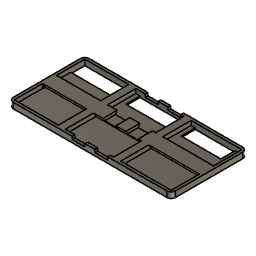
Top Side Cover 3x1 v5 (Autodesk Fusion 360 design; units mm, degrees)
Autodesk Fusion 360 part; units mm, degrees
sketch "Schizzo1" plane through (0, 0, 0) normal (0, 0, 1) x (1, 0, 0)
  line L0 (4.5367, 58.7959) -> (119.2367, 58.7959) construction
  line L1 (119.2367, 58.7959) -> (119.2367, 5.0959) construction
  line L2 (119.2367, 5.0959) -> (4.5367, 5.0959) construction
  line L3 (4.5367, 5.0959) -> (4.5367, 58.7959) construction
  line L4 (4.5367, 31.9459) -> (119.2367, 31.9459) construction
  line L5 (61.8867, 58.7959) -> (61.8867, 5.0959) construction
  line L6 (119.1367, 5.1959) -> (4.6367, 5.1959)
  line L7 (4.6367, 5.1959) -> (4.6367, 58.6959)
  line L8 (4.6367, 58.6959) -> (119.1367, 58.6959)
  line L9 (119.1367, 58.6959) -> (119.1367, 5.1959)
  line L10 (117.2367, 7.0959) -> (6.5367, 7.0959)
  line L11 (6.5367, 7.0959) -> (6.5367, 56.7959)
  line L12 (6.5367, 56.7959) -> (117.2367, 56.7959)
  line L13 (117.2367, 56.7959) -> (117.2367, 7.0959)
  line L14 (6.5367, 56.7959) -> (34.5367, 56.7959)
  line L15 (34.5367, 56.7959) -> (34.5367, 46.7959)
  line L16 (34.5367, 46.7959) -> (6.5367, 46.7959)
  line L17 (6.5367, 46.7959) -> (6.5367, 56.7959)
  line L18 (73.5367, 56.7959) -> (73.5367, 46.7959)
  line L19 (73.5367, 46.7959) -> (45.5367, 46.7959)
  line L20 (45.5367, 46.7959) -> (45.5367, 56.7959)
  line L21 (45.5367, 56.7959) -> (73.5367, 56.7959)
  line L22 (4.5367, 36.9459) -> (119.1367, 36.9459)
  line L23 (4.5367, 26.9459) -> (119.1367, 26.9459)
  line L24 (61.8867, 58.7959) -> (61.8867, 5.0959)
  line L25 (112.5367, 56.7959) -> (112.5367, 46.7959)
  line L26 (112.5367, 46.7959) -> (84.5367, 46.7959)
  line L27 (84.5367, 46.7959) -> (84.5367, 56.7959)
  line L28 (84.5367, 56.7959) -> (112.5367, 56.7959)
  line L29 (37.5367, 58.7959) -> (37.5367, 5.0959)
  line L30 (42.5367, 58.7959) -> (42.5367, 5.0959)
  line L31 (76.5367, 58.7959) -> (76.5367, 5.0959)
  line L32 (81.5367, 58.6959) -> (81.5367, 5.0959)
  dimension "d1" = 114.7
  dimension "d2" = 53.7
  dimension "d3" = 0.1
  dimension "d6" = 2
  dimension "d7" = 28
  dimension "d8" = 10
  dimension "d11" = 39
  dimension "d12" = 0
  dimension "d15" = 10
  dimension "d38" = 5
  dimension "d39" = 3
  dimension "d40" = 5
  dimension "d41" = 3
  constraint horizontal L0
  constraint vertical L1
  constraint horizontal L2
  constraint vertical L3
  constraint midpoint L3 L4.start
  constraint midpoint L1 L4.end
  constraint midpoint L0 L5.start
  constraint midpoint L2 L5.end
  constraint horizontal L14
  constraint vertical L15
  constraint horizontal L16
  constraint vertical L17
  constraint coincident L3 L22.start
  constraint coincident L9 L22.end
  constraint perpendicular L9 L22
  constraint symmetric L4 L22.start L23.start
  constraint symmetric L4 L22.end L23.end
  constraint coincident L0 L29.start
  constraint coincident L2 L29.end
  constraint perpendicular L6 L29
  constraint coincident L0 L30.start
  constraint coincident L2 L30.end
  constraint perpendicular L6 L30
  constraint coincident L0 L31.start
  constraint coincident L2 L31.end
  constraint perpendicular L2 L31
  constraint coincident L8 L32.start
  constraint coincident L2 L32.end
  constraint perpendicular L6 L32
  measures "d1" distance of L1 L3
  measures "d2" distance of L0 L2
  measures "d7" distance of L11.end L14.end
  measures "d8" distance of L11.end L16.end
  measures "d15" distance of L22 L23
  measures "d38" distance of L29 L30
  measures "d39" distance of L20 L30
  measures "d40" distance of L31 L32
  measures "d41" distance of L18 L31
extrude "Estrusione1" add sketch "Schizzo1" along normal blind 1 contours L10 L13 L23 L32 | L10 L23 L31 L32 | L13 L22 L23 L32 | L10 L23 L24 L31 | L22 L23 L31 L32 | L12 L13 L22 L25 L26 L27 L32 | L10 L23 L24 L30 | L22 L23 L24 L31 | L12 L22 L31 L32 | L10 L23 L29 L30 | L22 L23 L24 L30 | L12 L18 L19 L22 L24 L31 | L10 L11 L23 L29 | L22 L23 L29 L30 | L12 L19 L20 L22 L24 L30 | L11 L22 L23 L29 | L12 L22 L29 L30 | L11 L12 L15 L16 L22 L29
extrude "Estrusione2" add sketch "Schizzo1" along normal blind 4 contours L6 L9 L10 L13 L23 L32 | L6 L10 L31 L32 | L9 L13 L22 L23 | L6 L10 L24 L31 | L8 L9 L12 L13 L22 L28 L32 | L13 L22 L23 L32 | L6 L10 L24 L30 | L22 L23 L31 L32 | L6 L10 L29 L30 | L22 L23 L24 L31 | L8 L12 L31 L32 | L6 L7 L10 L11 L23 L29 | L22 L23 L24 L30 | L8 L12 L21 L24 L31 | L22 L23 L29 L30 | L8 L12 L21 L24 L30 | L7 L11 L22 L23 | L11 L22 L23 L29 | L8 L12 L29 L30 | L7 L8 L11 L12 L14 L17 L22 L29
fillet "Raccordo1" radius 3 4 edges at (4.6367, 5.1959, 2) (119.1367, 5.1959, 2) (119.1367, 58.6959, 2) (4.6367, 58.6959, 2)
ref_plane "Piano di lavoro1" through (61.8867, 31.9459, 0) normal (-1, 0, 0) x (0, -1, 0)
sketch "Schizzo3" plane through (61.8867, 0, 0) normal (-1, 0, 0) x (0, -1, 0)
  line L0 (-26.9459, 4) -> (-36.9459, 4) construction
  line L1 (-36.9459, 4) -> (-36.9459, 0) construction
  line L2 (-36.9459, 0) -> (-26.9459, 0) construction
  line L3 (-26.9459, 0) -> (-26.9459, 4) construction
  line L4 (-55.6959, 4) -> (-8.1959, 4) construction
  line L5 (-58.7959, 0) -> (-5.0959, 0) construction
  line L6 (-26.9459, 1) -> (-26.9459, 4) construction
  line L7 (-36.9459, 1) -> (-36.9459, 4) construction
  line L8 (-31.9459, 4) -> (-31.9459, 0) construction
  line L9 (-26.9459, 1) -> (-36.9459, 1) construction
  line L10 (-26.9459, 1) -> (-26.9459, 4)
  line L11 (-26.9459, 4) -> (-28.678, 1)
  line L12 (-28.678, 1) -> (-26.9459, 1)
  line L13 (-36.9459, 1) -> (-36.9459, 4)
  line L14 (-36.9459, 4) -> (-35.2139, 1)
  line L15 (-35.2139, 1) -> (-36.9459, 1)
  dimension "d20" = 30
  constraint horizontal L0
  constraint vertical L1
  constraint horizontal L2
  constraint vertical L3
  constraint collinear L0 L4
  constraint collinear L2 L5
  constraint collinear L3 L6
  constraint collinear L1 L7
  constraint midpoint L4 L8.start
  constraint midpoint L5 L8.end
  constraint coincident L6.start L9.start
  constraint coincident L7.start L9.end
  constraint coincident L0.start L3.end
  constraint coincident L9 L11.end
  constraint symmetric L8 L6.start L7.start
  constraint symmetric L8 L0.start L0.end
  constraint symmetric L8 L11.end L14.end
  measures "d20" angle of L10 L11
extrude "Estrusione4" cut sketch "Schizzo3" along normal mid plane 110
sketch "Schizzo4" plane through (0, 0, 4) normal (0, 0, 1) x (-1, 0, 0)
  arc A0 (-7.6367, -58.6959) -> (-4.6367, -55.6959) centre (-7.6367, -55.6959) ccw
  line L0 (-4.6367, -55.6959) -> (-4.6367, -8.1959)
  arc A1 (-4.6367, -8.1959) -> (-7.6367, -5.1959) centre (-7.6367, -8.1959) ccw
  line L1 (-7.6367, -5.1959) -> (-116.1367, -5.1959)
  arc A2 (-116.1367, -5.1959) -> (-119.1367, -8.1959) centre (-116.1367, -8.1959) ccw
  line L2 (-119.1367, -8.1959) -> (-119.1367, -55.6959)
  arc A3 (-119.1367, -55.6959) -> (-116.1367, -58.6959) centre (-116.1367, -55.6959) ccw
  line L3 (-116.1367, -58.6959) -> (-7.6367, -58.6959)
  line L4 (-117.2367, -36.9459) -> (-116.8867, -36.9459)
  line L5 (-116.8867, -36.9459) -> (-6.8867, -36.9459)
  line L6 (-6.8867, -36.9459) -> (-6.5367, -36.9459)
  line L7 (-6.5367, -36.9459) -> (-6.5367, -56.7959)
  line L8 (-6.5367, -56.7959) -> (-117.2367, -56.7959)
  line L9 (-117.2367, -56.7959) -> (-117.2367, -36.9459)
  line L10 (-117.2367, -7.0959) -> (-6.5367, -7.0959)
  line L11 (-6.5367, -7.0959) -> (-6.5367, -26.9459)
  line L12 (-6.5367, -26.9459) -> (-6.8867, -26.9459)
  line L13 (-6.8867, -26.9459) -> (-116.8867, -26.9459)
  line L14 (-117.2367, -26.9459) -> (-117.2367, -7.0959)
  line L15 (-4.6367, -58.6959) -> (-119.1367, -58.6959) construction
  line L16 (-119.1367, -58.6959) -> (-119.1367, -5.1959) construction
  line L17 (-119.1367, -5.1959) -> (-4.6367, -5.1959) construction
  line L18 (-4.6367, -5.1959) -> (-4.6367, -58.6959) construction
  line L19 (-49.2367, -58.6959) -> (-58.2367, -58.6959)
  line L20 (-58.2367, -58.6959) -> (-58.2367, -5.1959)
  line L21 (-58.2367, -5.1959) -> (-49.2367, -5.1959)
  line L22 (-49.2367, -5.1959) -> (-49.2367, -58.6959)
  line L23 (-65.2367, -58.6959) -> (-74.2367, -58.6959)
  line L24 (-74.2367, -58.6959) -> (-74.2367, -5.1959)
  line L25 (-74.2367, -5.1959) -> (-65.2367, -5.1959)
  line L26 (-65.2367, -5.1959) -> (-65.2367, -58.6959)
  line L27 (-53.7367, -58.6959) -> (-53.7367, -5.1959) construction
  line L28 (-69.7367, -58.6959) -> (-69.7367, -5.1959) construction
  line L29 (-2.7367, -58.6959) -> (-2.7367, -5.1959) construction
  line L30 (-116.8867, -26.9459) -> (-117.2367, -26.9459)
  dimension "d28" = 9
  dimension "d29" = 9
  dimension "d33" = 1.9
  dimension "d34" = 51
  dimension "d35" = 67
  constraint horizontal L15
  constraint vertical L16
  constraint horizontal L17
  constraint vertical L18
  constraint collinear L3 L15
  constraint collinear L0 L18
  constraint collinear L1 L17
  constraint collinear L2 L16
  constraint horizontal L19
  constraint vertical L20
  constraint horizontal L21
  constraint vertical L22
  constraint coincident L17 L20.end
  constraint coincident L15 L19.start
  constraint horizontal L23
  constraint vertical L24
  constraint horizontal L25
  constraint vertical L26
  constraint coincident L17 L24.end
  constraint coincident L3 L23.start
  constraint midpoint L19 L27.start
  constraint midpoint L21 L27.end
  constraint midpoint L23 L28.start
  constraint midpoint L25 L28.end
  constraint perpendicular L8 L29
  constraint coincident L15 L29.start
  constraint coincident L17 L29.end
  measures "d28" distance of L20 L22
  measures "d29" distance of L24 L26
  measures "d33" distance of L18 L29
  measures "d34" distance of L27 L29
  measures "d35" distance of L28 L29
extrude "Estrusione6" cut sketch "Schizzo4" against normal blind 2 contours L3 L8 L19 L20 L22 | L5 L8 L20 L22 | L3 L8 L23 L24 L26 | L5 L13 L20 L22 | L1 L10 L20 L21 L22 | L5 L8 L24 L26 | L10 L13 L20 L22 | L5 L13 L24 L26 | L1 L10 L24 L25 L26 | L10 L13 L24 L26
extrude "Estrusione7" add sketch "Schizzo1" along normal blind 4 contours L10 L23 L31 L32 | L22 L23 L31 L32 | L12 L22 L31 L32 | L10 L23 L29 L30 | L22 L23 L29 L30 | L12 L22 L29 L30
